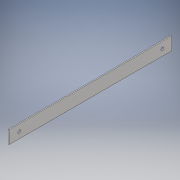
# Autodesk Inventor part: Platte_Kettenglied_oben
Saved by Autodesk Inventor 2018 (Build 220112000, 112)
## iProperties
Created: 2018-01-12
Part Number: Platte_Kettenglied_oben
Material: Generisch
Document SubType Name: Modeling
Designer: Julian
Density: 1 g/cm^3
Appearance: Vorgabe
Author: Julian
Autodesk Inventor part; units mm, degrees
ref_plane "YZ Plane" through (0, 0, 0) normal (1, 0, 0) x (0, 1, 0)
ref_plane "XZ Plane" through (0, 0, 0) normal (0, 1, 0) x (-1, 0, 0)
ref_plane "XY Plane" through (0, 0, 0) normal (0, 0, 1) x (1, 0, 0)
sketch "Skizze1" plane through (0, 0, 0) normal (1, 0, 0) x (0, 1, 0)
  line L0 (0, 0) -> (161.813, 0)
  line L1 (161.813, 0) -> (161.813, 12.7)
  line L2 (161.813, 12.7) -> (0, 12.7)
  line L3 (0, 12.7) -> (0, 0)
  dimension "d0" = 161.813
  dimension "d1" = 12.7
  constraints: 8 end point, 2 parallel, 1 horizontal, 1 perpendicular
  measures "d0" distance of L1.end L2.end
  measures "d1" distance of L2.end L0.start
extrude "Extrusion1" add sketch "Skizze1" along normal blind 1
sketch "Skizze2" plane through (1, 0, 0) normal (1, 0, 0) x (0, 0, -1)
  line L0 (-12.7, 0) -> (0, 0) projected
  line L1 (-6.35, 0) -> (-6.35, 10)
  line L2 (-6.35, 162.3865) -> (-6.35, 152.3865)
  dimension "d4" = 10
  dimension "d5" = 10
  constraints: 4 end point, 2 vertical, 1 midpoint
  measures "d4" distance of L1.start L1.end
  measures "d5" distance of L2.start L2.end
hole "Bohrung1" at (1, 10, 6.35) at (1, 152.3865, 6.35) direction (-1, 0, 0) diameter 3 end through all
